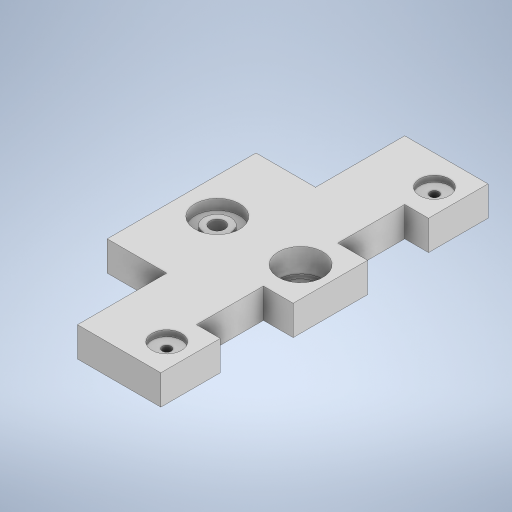
# Autodesk Inventor part: top
Saved by Autodesk Inventor 2023 (Build 270158000, 158)
## iProperties
Created: 2023-11-16
Part Number: top
Material: Všeobecné
Document SubType Name: Modeling
Designer: zavrel
Density: 1 g/cm^3
Appearance: Výchozí
Author: zavrel
Autodesk Inventor part; units mm, degrees
ref_plane "YZ Plane" through (0, 0, 0) normal (1, 0, 0) x (0, 1, 0)
ref_plane "XZ Plane" through (0, 0, 0) normal (0, 1, 0) x (-1, 0, 0)
ref_plane "XY Plane" through (0, 0, 0) normal (0, 0, 1) x (1, 0, 0)
sketch "Náčrt1" plane through (0, 0, 0) normal (0, 1, 0) x (-1, 0, 0)
  line L0 (-26.1298, 2.5) -> (-26.1298, 15)
  line L1 (-26.1298, 15) -> (-16.1298, 15)
  line L2 (-16.1298, 15) -> (-16.1298, 37.5)
  line L3 (-16.1298, 37.5) -> (-24.1298, 37.5)
  line L4 (-24.1298, 37.5) -> (-24.1298, 57.5)
  line L5 (-24.1298, 57.5) -> (-16.1298, 57.5)
  line L6 (-16.1298, 57.5) -> (3.8702, 57.5)
  line L7 (3.8702, 57.5) -> (3.8702, 27.5)
  line L8 (3.8702, 27.5) -> (23.8702, 27.5)
  line L9 (23.8702, 27.5) -> (23.8702, 2.5)
  line L10 (23.8702, 2.5) -> (-26.1298, 2.5) construction
  line L11 (-26.1298, 2.5) -> (-26.1298, -10)
  line L12 (-26.1298, -10) -> (-16.1298, -10)
  line L13 (-16.1298, -10) -> (-16.1298, -32.5)
  line L14 (-16.1298, -32.5) -> (-24.1298, -32.5)
  line L15 (-24.1298, -32.5) -> (-24.1298, -52.5)
  line L16 (-24.1298, -52.5) -> (-16.1298, -52.5)
  line L17 (-16.1298, -52.5) -> (3.8702, -52.5)
  line L18 (3.8702, -52.5) -> (3.8702, -22.5)
  line L19 (3.8702, -22.5) -> (23.8702, -22.5)
  line L20 (23.8702, -22.5) -> (23.8702, 2.5)
  circle A0 centre (-16.1298, 47.5) radius 5
  line L21 (-24.1298, 47.5) -> (17.4251, 47.5) construction
  circle A1 centre (-16.1298, -42.5) radius 5
  line L22 (-24.1298, -42.5) -> (17.4251, -42.5) construction
  circle A2 centre (11.8702, 2.5) radius 7.5
  circle A3 centre (-16.1298, 2.5) radius 7.5
  line L23 (-16.1298, 47.5) -> (-16.1298, -42.5) construction
  point P0 (0, 0)
  point P1 (-26.1298, 8.75)
  point P2 (-16.1298, 2.5)
  dimension "d0" = 25
  dimension "d1" = 50
  dimension "d3" = 20
  dimension "d4" = 8
  dimension "d5" = 20
  dimension "d6" = 20
  dimension "d7" = 10
  dimension "d8" = 90
  dimension "d9" = 8
  dimension "d10" = 15
  dimension "d13" = 15
  dimension "d15" = 12
  dimension "d17" = 10
  constraints: 48 end point, 12 symmetric about line, 9 perpendicular, 8 point on line, 4 centre point, 4 midpoint, 2 vertical, 1 horizontal, 1 other
  measures "d0" distance between parallel lines of L12 L1
  measures "d1" distance between parallel lines of L19 L8
  measures "d3" distance of L3.end L4.end
  measures "d4" distance between parallel lines of L13 L15
  measures "d5" distance between parallel lines of L13 L18
  measures "d6" distance between parallel lines of L18 L20
  measures "d7" diameter of A0
  measures "d8" distance of L23.end L23.start
  measures "d9" distance from line of L4 L23.start
  measures "d10" diameter of A2
  measures "d13" diameter of A3
  measures "d15" distance from line of L9 A2.centre
  measures "d17" distance of L11.end L12.end
extrude "Vysunutí1" add sketch "Náčrt1" along normal blind 10
sketch "Náčrt2" plane through (0, 0, 0) normal (0, -1, 0) x (1, 0, 0)
  line L0 (16.1298, -10) -> (16.1298, -32.5) projected
  line L1 (26.1298, -10) -> (16.1298, -10) projected
  line L2 (26.1298, 15) -> (26.1298, -10) projected
  line L3 (16.1298, 15) -> (26.1298, 15) projected
  line L4 (16.1298, 37.5) -> (16.1298, 15) projected
  line L5 (24.1298, 37.5) -> (16.1298, 37.5) projected
  line L6 (24.1298, 57.5) -> (24.1298, 37.5) projected
  line L7 (-3.8702, 57.5) -> (24.1298, 57.5) projected
  line L8 (-3.8702, 27.5) -> (-3.8702, 57.5) projected
  line L9 (-23.8702, 27.5) -> (-3.8702, 27.5) projected
  line L10 (-23.8702, -22.5) -> (-23.8702, 27.5) projected
  line L11 (-3.8702, -22.5) -> (-23.8702, -22.5) projected
  line L12 (-3.8702, -52.5) -> (-3.8702, -22.5) projected
  line L13 (24.1298, -52.5) -> (-3.8702, -52.5) projected
  line L14 (24.1298, -32.5) -> (24.1298, -52.5) projected
  line L15 (16.1298, -32.5) -> (24.1298, -32.5) projected
  circle A0 centre (16.1298, 47.5) radius 5 projected
  circle A1 centre (16.1298, -42.5) radius 5 projected
  circle A2 centre (-11.8702, 2.5) radius 7.5 projected
  circle A3 centre (16.1298, 2.5) radius 7.5 projected
  circle A4 centre (16.1298, -42.5) radius 1.5
  circle A5 centre (16.1298, 47.5) radius 5 projected
  circle A6 centre (16.1298, 47.5) radius 1.5
  point P0 (0, 0)
  dimension "d20" = 3
  constraints: 2 centre point, 2 coincident, 1 equal radius
  measures "d20" diameter of A6
extrude "Vysunutí2" add sketch "Náčrt2" against normal blind 8 contours A0 | A1
sketch "Náčrt3" plane through (0, 0, 0) normal (0, -1, 0) x (1, 0, 0)
  circle A0 centre (16.1298, 47.5) radius 1.5 projected
  circle A1 centre (16.1298, -42.5) radius 1.5 projected
  line L0 (16.1298, -10) -> (16.1298, -32.5) projected
  line L1 (26.1298, -10) -> (16.1298, -10) projected
  line L2 (26.1298, 15) -> (26.1298, -10) projected
  line L3 (16.1298, 15) -> (26.1298, 15) projected
  line L4 (16.1298, 37.5) -> (16.1298, 15) projected
  line L5 (24.1298, 37.5) -> (16.1298, 37.5) projected
  line L6 (24.1298, 57.5) -> (24.1298, 37.5) projected
  line L7 (-3.8702, 57.5) -> (24.1298, 57.5) projected
  line L8 (-3.8702, 27.5) -> (-3.8702, 57.5) projected
  line L9 (-23.8702, 27.5) -> (-3.8702, 27.5) projected
  line L10 (-23.8702, -22.5) -> (-23.8702, 27.5) projected
  line L11 (-3.8702, -22.5) -> (-23.8702, -22.5) projected
  line L12 (-3.8702, -52.5) -> (-3.8702, -22.5) projected
  line L13 (24.1298, -52.5) -> (-3.8702, -52.5) projected
  line L14 (24.1298, -32.5) -> (24.1298, -52.5) projected
  line L15 (16.1298, -32.5) -> (24.1298, -32.5) projected
  circle A2 centre (-11.8702, 2.5) radius 7.5 projected
  circle A3 centre (16.1298, 2.5) radius 7.5 projected
  circle A4 centre (16.1298, 2.5) radius 5.5
  point P0 (0, 0)
  dimension "d24" = 11
  constraints: 1 centre point, 1 coincident
  measures "d24" diameter of A4
extrude "Vysunutí3" add sketch "Náčrt3" against normal blind 2 contours A3
sketch "Náčrt4" plane through (0, 0, 0) normal (0, -1, 0) x (1, 0, 0)
  circle A0 centre (16.1298, 2.5) radius 5.5 projected
  circle A1 centre (16.1298, 47.5) radius 1.5 projected
  circle A2 centre (16.1298, -42.5) radius 1.5 projected
  line L0 (16.1298, -10) -> (16.1298, -32.5) projected
  line L1 (26.1298, -10) -> (16.1298, -10) projected
  line L2 (26.1298, 15) -> (26.1298, -10) projected
  line L3 (16.1298, 15) -> (26.1298, 15) projected
  line L4 (16.1298, 37.5) -> (16.1298, 15) projected
  line L5 (24.1298, 37.5) -> (16.1298, 37.5) projected
  line L6 (24.1298, 57.5) -> (24.1298, 37.5) projected
  line L7 (-3.8702, 57.5) -> (24.1298, 57.5) projected
  line L8 (-3.8702, 27.5) -> (-3.8702, 57.5) projected
  line L9 (-23.8702, 27.5) -> (-3.8702, 27.5) projected
  line L10 (-23.8702, -22.5) -> (-23.8702, 27.5) projected
  line L11 (-3.8702, -22.5) -> (-23.8702, -22.5) projected
  line L12 (-3.8702, -52.5) -> (-3.8702, -22.5) projected
  line L13 (24.1298, -52.5) -> (-3.8702, -52.5) projected
  line L14 (24.1298, -32.5) -> (24.1298, -52.5) projected
  line L15 (16.1298, -32.5) -> (24.1298, -32.5) projected
  circle A3 centre (-11.8702, 2.5) radius 7.5 projected
  circle A4 centre (-11.8702, 2.5) radius 2.5
  point P0 (0, 0)
  dimension "d27" = 5
  constraints: 1 centre point, 1 coincident
  measures "d27" diameter of A4
extrude "Vysunutí4" add sketch "Náčrt4" against normal blind 7.5 contours A3
sketch "Náčrt5" plane through (-11.8702, 7.5, 2.5) normal (0, 1, 0) x (1, 0, 0)
  circle A0 centre (0, 0) radius 7.5 projected
  circle A1 centre (0, 0) radius 2.5 projected
  circle A2 centre (0, 0) radius 2.5 projected
  circle A3 centre (0, 0) radius 4.5
  point P0 (11.8702, 2.5)
  dimension "d30" = 2
  constraints: 1 centre point, 1 coincident
  measures "d30" radial gap between concentric circles of A1 A3
extrude "Vysunutí5" cut sketch "Náčrt5" against normal blind 1 contours A0
